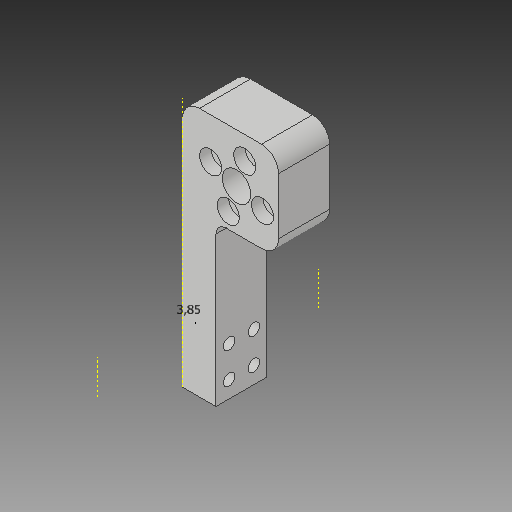
# Autodesk Inventor part: ZnutBracket
Saved by Autodesk Inventor 2019 (Build 230136000, 136)
## iProperties
Created: 2018-10-03
Part Number: ZnutBracket
Material: Generic
Document SubType Name: Modeling
Designer: LillaHunden
Density: 1 g/cm^3
Appearance: Default
Mass: 15.5939 g
Surface Area: 68.0106 cm^2
Volume: 15.5939 cm^3
Author: LillaHunden
Autodesk Inventor part; units mm, degrees
ref_plane "YZ Plane" through (0, 0, 0) normal (1, 0, 0) x (0, 1, 0)
ref_plane "XZ Plane" through (0, 0, 0) normal (0, 1, 0) x (-1, 0, 0)
ref_plane "XY Plane" through (0, 0, 0) normal (0, 0, 1) x (1, 0, 0)
sketch "Sketch1" plane through (0, 0, 0) normal (0, 0, 1) x (1, 0, 0)
  line L0 (-7.75, 8.5) -> (-7.75, 35.0829)
  line L1 (-7.75, 35.0829) -> (-36, 35.0829)
  line L2 (-36, 35.0829) -> (-36, -38.4359)
  line L3 (-36, -38.4359) -> (-20.05, -38.4359)
  line L4 (-20.05, -38.4359) -> (-20.05, -7.832)
  line L5 (-20.05, -7.832) -> (-26, -7.832)
  line L6 (-26, -7.832) -> (-26, 8.5)
  line L7 (-26, 8.5) -> (-7.75, 8.5)
  line L8 (6, -5.5) -> (6, -7.5) construction
  line L9 (6, -7.5) -> (25, -7.5) construction
  line L10 (25, -7.5) -> (25, 7.5) construction
  line L11 (25, 7.5) -> (7.55, 7.5) construction
  line L12 (7.55, 7.5) -> (7.55, 2.5) construction
  line L13 (7.55, 2.5) -> (-7.55, 2.5) construction
  line L14 (-7.55, 2.5) -> (-7.55, 7.5) construction
  line L15 (-7.55, 7.5) -> (-25, 7.5) construction
  line L16 (-25, 7.5) -> (-25, -7.5) construction
  line L17 (-25, -7.5) -> (-6, -7.5) construction
  line L18 (-6, -7.5) -> (-6, -5.5) construction
  line L19 (-6, -5.5) -> (6, -5.5) construction
  line L20 (-7.45, 2.5) -> (-7.45, 35.7282) construction
  line L21 (7.55, 2.5) -> (-7.45, 2.5) construction
  line L22 (7.55, 2.5) -> (7.55, 35.7282) construction
  line L23 (17.025, -18.5) -> (-20, -18.5) construction
  line L24 (-20, -18.5) -> (-20, -28.5) construction
  line L25 (17.025, -28.5) -> (-20, -28.5) construction
  line L26 (17.025, -18.5) -> (17.025, -28.5) construction
  line L27 (296.5, -28.5) -> (282.6818, -28.5) construction
  line L28 (296.5, -38.5) -> (282.6818, -38.5) construction
  circle A0 centre (15, 0) radius 1.621 projected
  circle A1 centre (-15, 0) radius 1.621 projected
  line L29 (7.55, 35.7282) -> (-7.45, 35.7282) projected
  circle A2 centre (0.0605, 28) radius 1.621 projected
  circle A3 centre (0.0605, 8) radius 1.621 projected
  line L30 (282.6818, -38.5) -> (282.6818, -28.5) projected
  line L31 (296.5, -28.5) -> (296.5, -38.5) projected
  point P0 (0, 0)
  dimension "d5" = 1
  dimension "d6" = 1
  dimension "d7" = 0.3
  dimension "d8" = 10
  constraints: 16 end point, 7 perpendicular, 1 vertical
  measures "d5" distance between parallel lines of L16 L6
  measures "d6" distance between parallel lines of L15 L7
  measures "d7" distance between parallel lines of L20 L0
  measures "d8" distance between parallel lines of L6 L2
extrude "Extrusion1" add sketch "Sketch1" along normal blind 15 contours L7 L6 L5 L4 L3 L2 L1 L0
sketch "Sketch2" plane through (0, 0, 15) normal (0, 0, 1) x (1, 0, 0)
  circle A0 centre (-20.1, 20.7) radius 5.15 construction
  circle A1 centre (-20.1, 20.7) radius 4.2
  point P0 (0, 0)
  dimension "d18" = 8.4
  constraints: 1 centre point
  measures "d18" diameter of A1
extrude "Extrusion2" cut sketch "Sketch2" against normal through all
sketch "Sketch3" plane through (-36, -38.4359, 0) normal (-1, 0, 0) x (0, 0, 1)
  line L0 (-25, 9.9359) -> (-25, -0.0641) construction
  line L1 (40, 19.9359) -> (40, 9.9359) construction
  line L2 (0, 0) -> (15, 0) construction
  line L3 (7.5, 0) -> (7.5, 20.6038) construction
  line L4 (15, 73.5188) -> (15, 0) construction
  point P0 (0, 38.4359)
  point P1 (11.1484, 4.9359)
  point P2 (3.8516, 4.9359)
  point P3 (11.15, 14.1056)
  point P4 (3.85, 14.1056)
  dimension "d10" = 3.85
  constraints: 2 end point, 2 symmetric about line, 1 midpoint, 1 vertical
  measures "d10" distance from line of L4 point (11.15, 14.106)
sketch "Sketch8" plane through (-36, 35.0829, 0) normal (-1, 0, 0) x (0, 0, 1)
  circle A0 centre (32.5096, -69.8259) radius 2.5 construction
  circle A1 centre (32.5096, -69.8259) radius 3.5
  point P0 (0, -35.0829)
  dimension "d28" = 7
  constraints: 1 centre point, 1 coincident
  measures "d28" diameter of A1
sketch "Sketch9" plane through (-36, 35.0829, 0) normal (-1, 0, 0) x (0, 0, 1)
  circle A0 centre (32.5096, -69.8259) radius 3.5 projected
  circle A1 centre (32.5096, -69.8259) radius 10
  point P0 (0, -35.0829)
  dimension "d31" = 20
  constraints: 1 centre point, 1 coincident
  measures "d31" diameter of A1
sketch "Sketch10" plane through (-36, 35.0829, 0) normal (-1, 0, 0) x (0, 0, 1)
  line L0 (45.4011, -39.3798) -> (15, -39.3798) projected
  line L1 (45.4011, -39.3798) -> (104.8234, -39.3798)
  line L2 (104.8234, -39.3798) -> (104.8234, -112.1071)
  line L3 (104.8234, -112.1071) -> (45.4011, -112.1071)
  line L4 (45.4011, -112.1071) -> (45.4011, -39.3798)
  line L5 (0, 0) -> (0, -81.2089) projected
  line L6 (0, -81.2089) -> (45.4011, -81.2089)
  line L7 (45.4011, -81.2089) -> (45.4011, -112.1071)
  line L8 (45.4011, -112.1071) -> (0, -112.1071)
  line L9 (0, -112.1071) -> (0, -81.2089)
  point P0 (0, -35.0829)
  constraints: 16 end point, 4 parallel, 2 horizontal, 2 perpendicular
sketch "Sketch11" plane through (-36, 35.0829, 0) normal (-1, 0, 0) x (0, 0, 1)
  circle A0 centre (96.9549, -98.5564) radius 2.5 construction
  circle A1 centre (96.9549, -51.4164) radius 2.75 construction
  circle A2 centre (49.8149, -98.5564) radius 2.5 construction
  circle A3 centre (49.8149, -51.4164) radius 2.75 construction
  circle A4 centre (96.9549, -98.5564) radius 2.75 construction
  circle A5 centre (96.9549, -51.4164) radius 2.5 construction
  point P0 (0, -35.0829)
sketch "Sketch12" plane through (-20.05, -7.832, 15) normal (1, 0, 0) x (0, 0, -1)
  line L0 (-86.5849, -8.3715) -> (-86.5849, -44.0215) construction
  line L1 (-30.1849, -55.7715) -> (-30.1849, -20.1215) construction
  arc A0 (-34.6849, -60.2715) -> (-30.1849, -55.7715) centre (-34.6849, -55.7715) ccw construction
  line L2 (-39.1849, -60.2715) -> (-34.6849, -60.2715) construction
  arc A1 (-30.4349, -8.3715) -> (-34.6849, -4.1215) centre (-34.6849, -8.3715) ccw construction
  line L3 (-30.4349, -8.3715) -> (-30.4349, -12.6215) construction
  line L4 (-30.4349, -12.6215) -> (-33.6849, -12.6215) construction
  arc A2 (-33.6849, -12.6215) -> (-33.6849, -20.1215) centre (-33.6849, -16.3715) ccw construction
  line L5 (-33.6849, -20.1215) -> (-30.4349, -20.1215) construction
  line L6 (-30.4349, -20.1215) -> (-30.4349, -55.7715) construction
  arc A3 (-34.6849, -60.0215) -> (-30.4349, -55.7715) centre (-34.6849, -55.7715) ccw construction
  line L7 (-34.6849, -60.0215) -> (-38.9349, -60.0215) construction
  line L8 (-38.9349, -60.0215) -> (-38.9349, -56.7715) construction
  arc A4 (-38.9349, -56.7715) -> (-46.4349, -56.7715) centre (-42.6849, -56.7715) ccw construction
  line L9 (-46.4349, -56.7715) -> (-46.4349, -60.0215) construction
  line L10 (-46.4349, -60.0215) -> (-82.0849, -60.0215) construction
  arc A5 (-86.3349, -55.7715) -> (-82.0849, -60.0215) centre (-82.0849, -55.7715) ccw construction
  line L11 (-86.3349, -55.7715) -> (-86.3349, -51.5215) construction
  line L12 (-86.3349, -51.5215) -> (-83.0849, -51.5215) construction
  arc A6 (-83.0849, -51.5215) -> (-83.0849, -44.0215) centre (-83.0849, -47.7715) ccw construction
  line L13 (-83.0849, -44.0215) -> (-86.3349, -44.0215) construction
  line L14 (-86.3349, -44.0215) -> (-86.3349, -8.3715) construction
  arc A7 (-82.0849, -4.1215) -> (-86.3349, -8.3715) centre (-82.0849, -8.3715) ccw construction
  line L15 (-82.0849, -4.1215) -> (-77.8349, -4.1215) construction
  line L16 (-77.8349, -4.1215) -> (-77.8349, -7.3715) construction
  arc A8 (-77.8349, -7.3715) -> (-70.3349, -7.3715) centre (-74.0849, -7.3715) ccw construction
  line L17 (-70.3349, -7.3715) -> (-70.3349, -4.1215) construction
  line L18 (-70.3349, -4.1215) -> (-34.6849, -4.1215) construction
  circle A9 centre (-81.9549, -55.6415) radius 2.75 construction
  circle A10 centre (-81.9549, -8.5015) radius 2.75 construction
  circle A11 centre (-34.8149, -8.5015) radius 2.75 construction
  circle A12 centre (-34.8149, -55.6415) radius 2.75 construction
  circle A13 centre (-58.3849, -32.0715) radius 19.3 construction
  line L19 (-89.8234, -69.1922) -> (-89.8234, 3.5351) projected
  line L20 (-89.8234, 3.5351) -> (0, 3.5351) projected
  line L21 (-89.8234, -69.1922) -> (-26.5432, -69.1922)
  line L22 (-26.5432, -69.1922) -> (-26.5432, 3.5351)
  line L23 (-26.5432, 3.5351) -> (-89.8234, 3.5351)
  line L24 (-89.8234, 3.5351) -> (-89.8234, -69.1922)
  point P0 (15, 7.832)
  constraints: 8 end point, 2 parallel, 1 horizontal, 1 perpendicular, 1 point on line
sketch "Sketch13" plane through (-20.05, -7.832, 15) normal (0, 0, -1) x (-1, 0, 0)
  line L0 (0, 0) -> (5.25, 0) projected
  line L1 (5.25, 0) -> (5.25, 3.5351) projected
  line L2 (5.25, 3.5351) -> (0, 3.5351) projected
  line L3 (0, 3.5351) -> (0, 0) projected
  point P0 (-20.05, 7.832)
sketch "Sketch14" plane through (-35.3, -77.0243, 104.8234) normal (0, 0, 1) x (1, 0, 0)
  line L0 (15.25, 69.1922) -> (10, 69.1922) projected
  line L1 (10, 69.1922) -> (15.25, 69.1922)
  line L2 (15.25, 69.1922) -> (15.25, 0)
  line L3 (15.25, 0) -> (10, 0)
  line L4 (10, 0) -> (10, 69.1922)
  point P0 (35.3, 77.0243)
  constraints: 8 end point, 2 parallel, 1 horizontal, 1 perpendicular
sketch "Sketch15" plane through (-30.05, -7.832, 15) normal (1, 0, 0) x (0, 0, -1)
  circle A0 centre (-58.3849, -32.0715) radius 19.3 construction
  circle A1 centre (-58.3849, -32.0715) radius 20.384
  point P0 (15, 7.832)
  constraints: 1 centre point
sketch "Sketch16" plane through (-31.05, -39.9036, 73.3849) normal (1, 0, 0) x (0, 0, -1)
  circle A0 centre (0, 0) radius 2.675 construction
  circle A1 centre (0, 0) radius 3.5
  point P0 (73.3849, 39.9036)
  dimension "d51" = 7
  constraints: 1 centre point, 1 coincident
  measures "d51" diameter of A1
sketch "Sketch4" plane through (-36, -38.4359, 0) normal (-1, 0, 0) x (0, 0, 1)
  point P0 (11.1484, 4.9359)
  point P1 (3.8516, 4.9359)
  point P2 (11.15, 14.1056)
  point P3 (3.85, 14.1056)
hole "Hole1" at (-36, -33.5, 11.1484) at (-36, -33.5, 3.8516) at (-36, -24.3303, 11.15) at (-36, -24.3303, 3.85) direction (1, 0, 0) diameter 3.4 depth 15.95 counterbore diameter 6.5 counterbore depth 3.4
sketch "Sketch6" plane through (0, 0, 15) normal (0, 0, 1) x (1, 0, 0)
  point P0 (-17.6836, 28.3263)
  point P1 (-12.4737, 18.2836)
  point P2 (-22.5164, 13.0737)
  point P3 (-27.7263, 23.1164)
hole "Hole3" at (-17.6836, 28.3263, 15) at (-12.4737, 18.2836, 15) at (-22.5164, 13.0737, 15) at (-27.7263, 23.1164, 15) direction (0, 0, -1) diameter 3.4 depth 15 counterbore diameter 6.5 counterbore depth 3.4
sketch "Sketch17" plane through (0, 0, 15) normal (0, 0, 1) x (1, 0, 0)
  line L0 (-36, -38.4359) -> (-20.05, -38.4359) projected
  line L1 (-20.05, -38.4359) -> (-20.05, -7.832) projected
  line L2 (-26.1554, -38.4359) -> (-20.05, -38.4359)
  line L3 (-20.05, -38.4359) -> (-20.05, 8.5)
  line L4 (-20.05, 8.5) -> (-26.1554, 8.5)
  line L5 (-26.1554, 8.5) -> (-26.1554, -38.4359)
  point P0 (0, 0)
  point P1 (-26, 8.5)
  constraints: 8 end point, 3 point on line, 2 parallel, 1 horizontal, 1 perpendicular
extrude "Extrusion12" cut sketch "Sketch17" against normal through all
fillet "Fillet1" radius 5 2 edges at (-36, 35.0829, 7.5) (-7.75, 35.0829, 7.5)
fillet "Fillet2" radius 5 1 edges at (-7.75, 8.5, 7.5)
fillet "Fillet3" radius 3 1 edges at (-26.1554, 8.5, 7.5)
body "Solid1"
